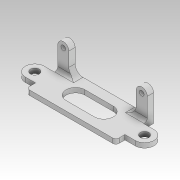
# Autodesk Inventor part: IntegzaBracket
Saved by Autodesk Inventor 2020 (Build 240168000, 168)
## iProperties
Created: 2022-01-26
Part Number: IntegzaBracket
Material: Generic
Document SubType Name: Modeling
Designer: DDeGo
Density: 1 g/cm^3
Appearance: Default
Author: DDeGo
Autodesk Inventor part; units mm, degrees
ref_plane "YZ Plane" through (0, 0, 0) normal (1, 0, 0) x (0, 1, 0)
ref_plane "XZ Plane" through (0, 0, 0) normal (0, 1, 0) x (-1, 0, 0)
ref_plane "XY Plane" through (0, 0, 0) normal (0, 0, 1) x (1, 0, 0)
sketch "Sketch1" plane through (0, 0, 0) normal (0, 0, 1) x (1, 0, 0)
  line L0 (0, 0) -> (-25, 0) construction
  line L1 (0, 0) -> (25, 0) construction
  circle A0 centre (-25, 0) radius 1.5
  circle A1 centre (25, 0) radius 1.5
  line L2 (-21.5, -14) -> (21.5, -14)
  line L3 (28.5, -11.1976) -> (28.5, -17)
  line L4 (28.5, -17) -> (-28.5, -17)
  line L5 (-28.5, -17) -> (-28.5, 0.6332)
  line L6 (-21.5, -14) -> (-21.5, 0)
  line L7 (-28.5, 0) -> (-28.5, 0.6332)
  line L8 (21.5, -14) -> (21.5, 0)
  line L9 (28.5, 0) -> (28.5, -11.1976)
  arc A2 (28.5, 0) -> (21.5, 0) centre (25, 0) ccw
  arc A3 (-21.5, 0) -> (-28.5, 0) centre (-25, 0) ccw
  dimension "d0" = 50
  dimension "d1" = 3
  dimension "d2" = 3.5
  dimension "d3" = 17
  dimension "d4" = 3
  constraints: 20 end point, 4 centre point, 4 coincident, 4 parallel, 4 point on circle, 4 tangent, 3 horizontal, 2 equal radius, 2 vertical, 1 collinear, 1 perpendicular
  measures "d0" distance of L1.end L0.end
  measures "d1" diameter of A0
  measures "d2" radius of A3
  measures "d3" distance between parallel lines of L4 L0
  measures "d4" distance between parallel lines of L4 L2
extrude "Extrusion1" add sketch "Sketch1" along normal blind 4
sketch "Sketch2" plane through (0, 0, 4) normal (0, 0, 1) x (1, 0, 0)
  line L0 (28.5, -17) -> (28.5, 0) projected
  line L1 (28.5, -17) -> (-28.5, -17)
  line L2 (-28.5, -17) -> (-28.5, -14)
  line L3 (-28.5, -14) -> (28.5, -14)
  line L4 (28.5, -14) -> (28.5, -17)
  line L5 (-28.5, 0) -> (-28.5, -17) projected
  point P0 (0, 0)
  point P1 (-21.5, -14)
  constraints: 8 end point, 2 parallel, 2 point on line, 1 horizontal, 1 perpendicular
extrude "Extrusion2" add sketch "Sketch2" along normal blind 20
sketch "Sketch3" plane through (-28.5, -17, 0) normal (0, -1, 0) x (1, 0, 0)
  line L0 (28.5, 0) -> (28.5, 12.2) construction
  line L1 (-6.5, 12.2) -> (63.5, 12.2) construction
  line L2 (0, 24) -> (57, 24) projected
  line L3 (-6.5, 6.2) -> (63.5, 6.2)
  line L4 (63.5, 18.2) -> (-6.5, 18.2)
  arc A0 (-6.5, 18.2) -> (-6.5, 6.2) centre (-6.5, 12.2) ccw
  arc A1 (63.5, 6.2) -> (63.5, 18.2) centre (63.5, 12.2) ccw
  line L5 (0, 4) -> (7, 4) projected
  circle A2 centre (-6.5, 12.2) radius 2.75
  circle A3 centre (63.5, 12.2) radius 2.75
  dimension "d9" = 6
  dimension "d10" = 70
  dimension "d11" = 8.2
  dimension "d12" = 5.5
  constraints: 10 end point, 4 centre point, 4 point on circle, 4 tangent, 2 coincident, 2 parallel, 1 equal radius, 1 midpoint, 1 vertical
  measures "d9" radius of A1
  measures "d10" distance of L1.start L1.end
  measures "d11" distance between parallel lines of L1 L5
  measures "d12" diameter of A2
extrude "Extrusion3" add sketch "Sketch3" against normal up to surface (3 mm away)
sketch "Sketch4" plane through (-21.5, -14, 0) normal (0, 1, 0) x (1, 0, 0)
  circle A0 centre (-13.5, -12.2) radius 2.75 construction
  line L0 (-13.5, -12.2) -> (21.5, -12.2) construction
  line L1 (21.5, -12.2) -> (21.5, 0) construction
  line L2 (-7, 0) -> (50, 0) construction
  line L3 (30.5, -12.2) -> (12.5, -12.2) construction
  line L4 (30.5, -6.2) -> (12.5, -6.2)
  line L5 (12.5, -18.2) -> (30.5, -18.2)
  arc A1 (30.5, -18.2) -> (30.5, -6.2) centre (30.5, -12.2) ccw
  arc A2 (12.5, -6.2) -> (12.5, -18.2) centre (12.5, -12.2) ccw
  dimension "d15" = 6
  dimension "d16" = 18
  constraints: 12 end point, 4 point on circle, 4 tangent, 2 centre point, 1 horizontal, 1 midpoint, 1 parallel, 1 perpendicular, 1 point on line
  measures "d15" radius of A2
  measures "d16" distance of L3.start L3.end
extrude "Extrusion4" cut sketch "Sketch4" against normal through all
fillet "Fillet1" radius 2 2 edges at (-28.5, -15.5, 24) (28.5, -15.5, 24)
fillet "Fillet2" radius 2 2 edges at (-25, -14, 4) (25, -14, 4)
fillet "Fillet3" radius 5 4 edges at (-21.5, -14, 5) (-21.5, -14, 2) (21.5, -14, 2) (21.5, -14, 5)
body "Solid1"
